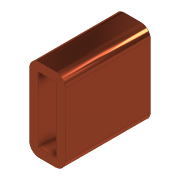
# Autodesk Inventor part: coil
Saved by Autodesk Inventor 2020 (Build 240168000, 168)
## iProperties
Created: 2020-05-19
Part Number: coil
Material: Generic
Document SubType Name: Modeling
Designer: Kostic
Density: 1 g/cm^3
Appearance: Copper - Polished
Author: Kostic
Autodesk Inventor part; units mm, degrees
ref_plane "YZ Plane" through (0, 0, 0) normal (1, 0, 0) x (0, 1, 0)
ref_plane "XZ Plane" through (0, 0, 0) normal (0, 1, 0) x (-1, 0, 0)
ref_plane "XY Plane" through (0, 0, 0) normal (0, 0, 1) x (1, 0, 0)
sketch "Sketch1" plane through (0, 0, 0) normal (0, 0, 1) x (1, 0, 0)
  line L0 (-1.1, 4) -> (1.1, 4)
  line L1 (1.1, 4) -> (1.1, -4)
  line L2 (1.1, -4) -> (-1.1, -4)
  line L3 (-1.1, -4) -> (-1.1, 4)
  line L4 (-2.2, 5.1) -> (2.2, 5.1)
  line L5 (2.2, 5.1) -> (2.2, -5.1)
  line L6 (2.2, -5.1) -> (-2.2, -5.1)
  line L7 (-2.2, -5.1) -> (-2.2, 5.1)
  point P0 (0, 0)
  dimension "d0" = 2.2
  dimension "d1" = 8
  dimension "d2" = 1.1
  dimension "d3" = 4
  dimension "d4" = 2.2
  dimension "d5" = 2.2
  dimension "d6" = 1.1
  dimension "d7" = 1.1
  dimension "d8" = 1.1
  constraints: 16 end point, 4 parallel, 2 horizontal, 2 perpendicular
  measures "d0" distance of L1.end L2.end
  measures "d1" distance of L0.end L1.end
  measures "d2" distance from line of L1 point (0, 0)
  measures "d3" distance from line of point (0, 0) L0
  measures "d4" distance from line of point (0, 0) L7
  measures "d5" distance from line of L5 point (0, 0)
  measures "d6" distance between parallel lines of L7 L3
  measures "d7" distance between parallel lines of L4 L0
  measures "d8" distance between parallel lines of L6 L2
extrude "Extrusion1" add sketch "Sketch1" along normal blind 10.5
fillet "Fillet1" radius 1.2 4 edges at (2.2, 5.1, 5.25) (-2.2, 5.1, 5.25) (-2.2, -5.1, 5.25) (2.2, -5.1, 5.25)
equation "\"d2\" = 0.5 * d0"
equation "\"d3\" = 0.5 * d1"
equation "\"d5\" = d4"
equation "\"d7\" = d6"
equation "\"d8\" = d6"
body "Solid1"
